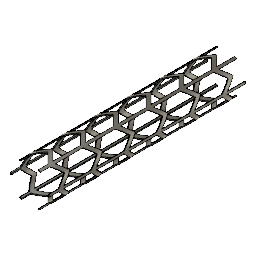
Stent2 (Autodesk Fusion 360 design; units mm, degrees)
Autodesk Fusion 360 part; units mm, degrees
sketch "Sketch1" plane through (0, 0, 0) normal (0, 0, 1) x (1, 0, 0)
  line L0 (0, 0) -> (0, 15) construction
  dimension "d1" = 15
  constraint coincident L0.start origin
  constraint vertical L0
  measures "d1" distance of L0.start L0.end
sketch "Sketch2" plane through (0, 0, 0) normal (0, 1, 0) x (1, 0, 0)
  circle A0 centre (0, 0) radius 1.4
  circle A1 centre (0, 0) radius 1.48
  line L0 (0, 0) -> (0, -1.48) construction
  dimension "d2" = 2.8
  dimension "d6" = 0.08
  constraint coincident A0.centre A1.centre
  constraint concentric A0 A1
  constraint coincident A1 L0.end
  constraint vertical L0
  measures "d2" diameter of A0
  measures "d6" distance of A0 A1
extrude "Extrude2" add sketch "Sketch2" along normal blind 15
sketch "Sketch4" plane through (0, 0, 0) normal (0, 0, 1) x (1, 0, 0)
  line L0 (1.48, 0) -> (1.48, 15)
  line L1 (-1.48, 15) -> (-1.48, 0)
  line L2 (1.48, 15) -> (-1.48, 15)
  line L3 (1.48, 0) -> (-1.48, 0)
  line L4 (-0.65, 0.725) -> (0, 1.375)
  line L5 (0, -0.725) -> (0, 1.375) construction
  line L6 (-0.65, 0.725) -> (-0.65, -1.375)
  line L7 (-0.65, -1.375) -> (0, -0.725)
  line L8 (0.65, 0.725) -> (0.65, -1.375)
  line L9 (0.65, -1.375) -> (0, -0.725)
  line L10 (0.65, 0.725) -> (0, 1.375)
  line L11 (-0.65, 1.125) -> (0, 1.775)
  line L12 (-0.65, 3.225) -> (-0.65, 1.125)
  line L13 (-0.65, 3.225) -> (0, 3.875)
  line L14 (0.65, 3.225) -> (0, 3.875)
  line L15 (0.65, 3.225) -> (0.65, 1.125)
  line L16 (0.65, 1.125) -> (0, 1.775)
  line L17 (-0.65, 3.625) -> (0, 4.275)
  line L18 (-0.65, 5.725) -> (-0.65, 3.625)
  line L19 (-0.65, 5.725) -> (0, 6.375)
  line L20 (0.65, 5.725) -> (0, 6.375)
  line L21 (0.65, 5.725) -> (0.65, 3.625)
  line L22 (0.65, 3.625) -> (0, 4.275)
  line L23 (-0.65, 6.125) -> (0, 6.775)
  line L24 (-0.65, 8.225) -> (-0.65, 6.125)
  line L25 (-0.65, 8.225) -> (0, 8.875)
  line L26 (0.65, 8.225) -> (0, 8.875)
  line L27 (0.65, 8.225) -> (0.65, 6.125)
  line L28 (0.65, 6.125) -> (0, 6.775)
  line L29 (-0.65, 8.625) -> (0, 9.275)
  line L30 (-0.65, 10.725) -> (-0.65, 8.625)
  line L31 (-0.65, 10.725) -> (0, 11.375)
  line L32 (0.65, 10.725) -> (0, 11.375)
  line L33 (0.65, 10.725) -> (0.65, 8.625)
  line L34 (0.65, 8.625) -> (0, 9.275)
  line L35 (-0.65, 11.125) -> (0, 11.775)
  line L36 (-0.65, 13.225) -> (-0.65, 11.125)
  line L37 (-0.65, 13.225) -> (0, 13.875)
  line L38 (0.65, 13.225) -> (0, 13.875)
  line L39 (0.65, 13.225) -> (0.65, 11.125)
  line L40 (0.65, 11.125) -> (0, 11.775)
  line L41 (-0.65, 13.625) -> (0, 14.275)
  line L42 (-0.65, 15.725) -> (-0.65, 13.625)
  line L43 (-0.65, 15.725) -> (0, 16.375)
  line L44 (0.65, 15.725) -> (0, 16.375)
  line L45 (0.65, 15.725) -> (0.65, 13.625)
  line L46 (0.65, 13.625) -> (0, 14.275)
  dimension "d41" = 2.1
  dimension "d42" = 1.375
  dimension "d43" = 0.725
  dimension "d44" = 45
  dimension "d45" = 0.65
  dimension "d48" = 0
  dimension "d49" = 15
  constraint vertical L5
  constraint vertical L6
  constraint parallel L4 L7
  constraint symmetric L4.start L5 L8.start
  constraint symmetric L4.end L5 L10.end
  constraint symmetric L7.end L5 L9.end
  constraint symmetric L6.end L5 L8.end
  measures "d41" distance of L4.end L5.start
  measures "d42" distance of origin L4.end
  measures "d43" distance of L3 L5.start
  measures "d44" angle of L6 L7
  measures "d45" distance of L5 L6
extrude "Extrude3" cut sketch "Sketch4" along normal through all contours L3 L6 L7 L8 L9 | L3 L4 L6 L8 L10 | L2 L41 L42 L45 L46 | L2 L42 L43 L44 L45 | L11 L12 L13 L14 L15 L16 | L17 L18 L19 L20 L21 L22 | L23 L24 L25 L26 L27 L28 | L29 L30 L31 L32 L33 L34 | L35 L36 L37 L38 L39 L40
pattern_circular "C-Pattern1" count 6 over 360 about axis through (0, -0.725, 0) along (0, 1, 0) of "Extrude3"
ref_plane "WorkPlane2" through (0, 0, 0) normal (0, 0, 1) x (1, 0, 0)
ref_plane "WorkPlane3" through (0, 7.5, 0) normal (0.5, 0, 0.866025) x (0, 1, 0)
